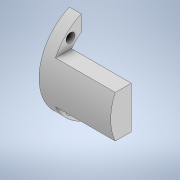
# Autodesk Inventor part: Lid_Tilt
Saved by Autodesk Inventor 2022 (Build 260153000, 153)
## iProperties
Created: 2022-04-03
Part Number: Lid_Tilt
Material: Generic
Document SubType Name: Modeling
Designer: Mlees
Density: 1 g/cm^3
Appearance: Default
Author: Mlees
Autodesk Inventor part; units mm, degrees
ref_plane "YZ Plane" through (0, 0, 0) normal (1, 0, 0) x (0, 1, 0)
ref_plane "XZ Plane" through (0, 0, 0) normal (0, 1, 0) x (-1, 0, 0)
ref_plane "XY Plane" through (0, 0, 0) normal (0, 0, 1) x (1, 0, 0)
sketch "Sketch1" plane through (0, 0, 0) normal (1, 0, 0) x (0, 1, 0)
  arc A0 (31.1103, 13.7167) -> (-31.1103, 13.7167) centre (0, 0) ccw
  arc A1 (20.4522, 13.7167) -> (-20.4522, 13.7167) centre (0, 0) ccw
  line L0 (0, 0) -> (34, 0) construction
  circle A2 centre (20.9487, 20.9487) radius 1.5
  line L1 (31.1103, 13.7167) -> (20.4522, 13.7167)
  line L2 (-20.4522, 13.7167) -> (-31.1103, 13.7167)
  line L3 (0, 0) -> (34, 0) construction
  circle A3 centre (-20.9487, 20.9487) radius 1.5
  constraints: 8 end point, 4 centre point, 4 horizontal, 4 point on circle, 2 coincident
extrude "Extrusion1" add sketch "Sketch1" along normal blind 8
sketch "Sketch2" plane through (8, 0, 0) normal (1, 0, 0) x (0, 0, -1)
  circle A0 centre (-20.9487, 20.9487) radius 1.5 projected
  circle A1 centre (-20.9487, 20.9487) radius 3
  circle A2 centre (-20.9487, -20.9487) radius 1.5 projected
  circle A3 centre (-20.9487, -20.9487) radius 3
  point P0 (0, 0)
  dimension "d8" = 6
  constraints: 2 centre point, 2 coincident
  measures "d8" diameter of A1
extrude "Extrusion2" cut sketch "Sketch2" against normal blind 4
sketch "Sketch3" plane through (8, 0, 0) normal (1, 0, 0) x (0, 0, -1)
  line L0 (-20.1744, 14.1221) -> (-30.9284, 14.1221)
  arc A0 (-13.7167, 31.1103) -> (-13.7167, -31.1103) centre (0, 0) ccw projected
  line L1 (-20.1744, -14.1221) -> (-30.9284, -14.1221)
  arc A1 (-30.9284, 14.1221) -> (-30.9284, -14.1221) centre (0, 0) ccw
  line L2 (-20.1744, 14.1221) -> (-20.1744, -14.1221)
  constraints: 6 end point, 4 point on circle, 1 centre point, 1 horizontal, 1 vertical
extrude "Extrusion3" add sketch "Sketch3" along normal blind 40
body "Solid1"
